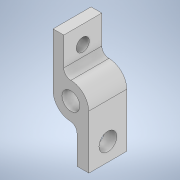
# Autodesk Inventor part: 15
Saved by Autodesk Inventor 2022 (Build 260153000, 153)
## iProperties
Created: 2022-03-14
Part Number: 15
Material: Všeobecné
Document SubType Name: Modeling
Designer: Šimon
Density: 1 g/cm^3
Appearance: Výchozí
Author: Šimon
Autodesk Inventor part; units mm, degrees
ref_plane "YZ Plane" through (0, 0, 0) normal (1, 0, 0) x (0, 1, 0)
ref_plane "XZ Plane" through (0, 0, 0) normal (0, 1, 0) x (-1, 0, 0)
ref_plane "XY Plane" through (0, 0, 0) normal (0, 0, 1) x (1, 0, 0)
sketch "Náčrt1" plane through (0, 0, 0) normal (0, 0, 1) x (1, 0, 0)
  line L0 (5.1631, -20.9413) -> (5.1631, -45)
  arc A0 (5.1631, -20.9413) -> (0, -15) centre (-0.8369, -20.9413) ccw
  line L1 (5.1631, -45) -> (15.1631, -45)
  line L2 (15.1631, -45) -> (14.9999, 0.0543)
  line L3 (-14.9999, 0.0543) -> (-14.9999, 45)
  arc A1 (-6, 21) -> (0, 15) centre (0, 21) ccw
  line L4 (-6, 21) -> (-6, 45)
  line L5 (-6, 45) -> (-14.9999, 45)
  circle A2 centre (0, 0) radius 7.5
  arc A3 (-14.9999, 0.0543) -> (0, -15) centre (0, 0) ccw
  arc A4 (14.9999, 0.0543) -> (0, 15) centre (0, 0) ccw
  dimension "d1" = 6
  dimension "d2" = 45
  dimension "d3" = 10
  dimension "d10" = 12
  dimension "d11" = 15
  constraints: 12 end point, 8 point on circle, 5 centre point, 3 tangent, 3 vertical, 2 coincident, 1 horizontal, 1 perpendicular
  measures "d1" radius of A0
  measures "d2" vertical distance of L0.end point (0, 0)
  measures "d3" distance of L0.end L1.end
  measures "d10" diameter of A1
  measures "d11" diameter of A2
extrude "Vysunutí1" add sketch "Náčrt1" along normal blind 32
sketch "Náčrt2" plane through (14.9999, 0.0543, 32) normal (1, 0.0036, 0) x (0, 0, -1)
  line L0 (32, -45.0184) -> (0, -45.0184) projected
  circle A0 centre (16, -30.0184) radius 7.5
  line L1 (32, -45.0546) -> (32, 0) projected
  dimension "d15" = 15
  dimension "d16" = 15
  dimension "d17" = 16
  constraints: 1 centre point
  measures "d15" diameter of A0
  measures "d16" distance from line of L0 A0.centre
  measures "d17" distance from line of L1 A0.centre
extrude "Vysunutí2" cut sketch "Náčrt2" against normal blind 32
sketch "Náčrt3" plane through (-6, 21, 0) normal (1, 0, 0) x (0, 0, -1)
  circle A0 centre (-16, 9) radius 5.4921
  line L0 (0, 0) -> (0, 24) projected
  line L1 (0, 24) -> (-32, 24) projected
  point P0 (0, -21)
  dimension "d20" = 16
  dimension "d21" = 15
  constraints: 1 centre point
  measures "d20" distance from line of L0 A0.centre
  measures "d21" distance from line of L1 A0.centre
extrude "Vysunutí3" cut sketch "Náčrt3" against normal blind 32
